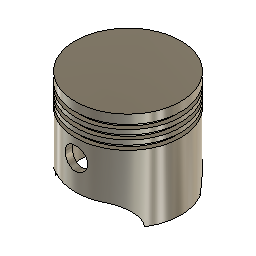
piston 3d (Autodesk Fusion 360 design; units mm, degrees)
Autodesk Fusion 360 part; units mm, degrees
sketch "Sketch1" plane through (0, 0, 0) normal (0, 1, 0) x (1, 0, 0)
  line L0 (0, 0) -> (0, -88)
  line L1 (0, -88) -> (47, -88)
  line L2 (47, -88) -> (47, -80)
  line L3 (47, -80) -> (43, -80)
  line L4 (43, -80) -> (43, -76)
  line L5 (43, -76) -> (47, -76)
  line L6 (47, -76) -> (47, -72)
  line L7 (47, -72) -> (43, -72)
  line L8 (43, -72) -> (43, -68)
  line L9 (43, -68) -> (47, -68)
  line L10 (47, -68) -> (47, -64)
  line L11 (47, -64) -> (43, -64)
  line L12 (43, -64) -> (43, -60)
  line L13 (43, -60) -> (47, -60)
  line L14 (47, -60) -> (47, -0.077)
  line L15 (47, -0.077) -> (41, -0.077)
  line L16 (41, -0.077) -> (41, -80)
  line L17 (41, -80) -> (0, -80)
  dimension "d1" = 88
  dimension "d2" = 47
  dimension "d3" = 8
  dimension "d4" = 4
  dimension "d5" = 4
  dimension "d6" = 4
  dimension "d7" = 4
  dimension "d8" = 4
  dimension "d9" = 4
  dimension "d10" = 4
  dimension "d11" = 4
  dimension "d12" = 4
  dimension "d13" = 4
  dimension "d14" = 4
  dimension "d16" = 6
  constraint coincident L0.start origin
  constraint vertical L0
  constraint perpendicular L0 L1
  constraint perpendicular L1 L2
  constraint perpendicular L2 L3
  constraint perpendicular L3 L4
  constraint perpendicular L4 L5
  constraint perpendicular L5 L6
  constraint perpendicular L4 L7
  constraint perpendicular L5 L8
  constraint perpendicular L8 L9
  constraint perpendicular L5 L10
  constraint perpendicular L8 L11
  constraint perpendicular L5 L12
  constraint perpendicular L8 L13
  constraint perpendicular L13 L14
  constraint perpendicular L14 L15
  constraint perpendicular L3 L16
  constraint coincident L0 L17.end
  constraint perpendicular L0 L17
  measures "d1" distance of L0.start L0.end
  measures "d2" distance of L0.end L1.end
  measures "d3" distance of L1.end L2.end
  measures "d4" distance of L2.end L3.end
  measures "d5" distance of L3.end L4.end
  measures "d6" distance of L4.end L5.end
  measures "d7" distance of L5.end L6.end
  measures "d8" distance of L6.end L7.end
  measures "d9" distance of L7.end L8.end
  measures "d10" distance of L8.end L9.end
  measures "d11" distance of L9.end L10.end
  measures "d12" distance of L10.end L11.end
  measures "d13" distance of L11.end L12.end
  measures "d14" distance of L12.end L13.end
  measures "d16" distance of L14.end L15.end
revolve "Revolve1" add sketch "Sketch1" angle 360 about axis through (0, 0, 0) along (0, 0, 1)
sketch "Sketch2" plane through (0, 0, 0) normal (0, 1, 0) x (1, 0, 0)
  line L0 (-46.9446, 0) -> (-39.667, 0)
  line L1 (-21.667, -18) -> (0, -18)
  line L2 (0, 0) -> (0, -37.5033) construction
  arc A0 (-39.667, 0) -> (-21.667, -18) centre (-21.667, 0) ccw
  line L3 (21.667, -18) -> (0, -18)
  arc A1 (21.667, -18) -> (39.667, 0) centre (21.667, 0) ccw
  circle A2 centre (0, -44) radius 10
  line L4 (-39.667, 0) -> (39.667, 0)
  point P0 (-39.667, -18)
  dimension "d17" = 18
  dimension "d18" = 18
  dimension "d19" = 20
  dimension "d20" = 44
  constraint horizontal L0
  constraint coincident L2.start origin
  constraint perpendicular L1 L2
  constraint coincident P0 L1
  constraint tangent L1 A0
  constraint coincident L0.end A0.start
  constraint symmetric L1.end L2 L3.end
  constraint symmetric L2 L1.start L3.start
  constraint symmetric L2 L0.end A1.end
  constraint symmetric L2 A0 A1
  constraint parallel L0 L4
  measures "d17" distance of L0.end P0
  measures "d18" radius of A0
  measures "d19" diameter of A2
  measures "d20" distance of L2.start A2.centre
extrude "Extrude1" cut sketch "Sketch2" along normal mid plane 180
